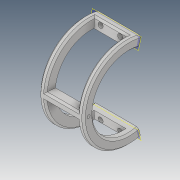
# Autodesk Inventor part: thrusterGuard2
Saved by Autodesk Inventor 2018 (Build 220112000, 112)
## iProperties
Created: 2020-01-11
Part Number: thrusterGuard2
Material: Generic
Document SubType Name: Modeling
Designer: anirudh
Density: 1 g/cm^3
Appearance: Default
Author: anirudh
Autodesk Inventor part; units mm, degrees
ref_plane "YZ Plane" through (0, 0, 0) normal (1, 0, 0) x (0, 1, 0)
ref_plane "XZ Plane" through (0, 0, 0) normal (0, 1, 0) x (-1, 0, 0)
ref_plane "XY Plane" through (0, 0, 0) normal (0, 0, 1) x (1, 0, 0)
sketch "Sketch1" plane through (0, 0, 0) normal (1, 0, 0) x (0, 1, 0)
  arc A0 (49.069, -13.148) -> (-49.069, -13.148) centre (0, 0) ccw
  arc A1 (62.7838, -16.8229) -> (-62.7838, -16.8229) centre (0, 0) ccw
  line L0 (49.069, -13.148) -> (62.7838, -16.8229)
  line L1 (0, 0) -> (80.3094, 0) construction
  line L2 (-49.069, -13.148) -> (-62.7838, -16.8229)
  line L3 (0, 0) -> (80.3094, 0) construction
  constraints: 8 end point, 4 point on circle, 2 centre point, 2 coincident, 2 horizontal
extrude "Extrusion1" add sketch "Sketch1" along normal blind 8.89
sketch "Sketch2" plane through (8.89, 0, 0) normal (1, 0, 0) x (0, 0, -1)
  line L0 (13.148, 49.069) -> (16.8229, 62.7838) projected
  line L1 (13.148, 49.069) -> (16.8229, 62.7838)
  arc A0 (16.8229, 62.7838) -> (16.8229, -62.7838) centre (0, 0) ccw projected
  line L2 (13.148, -49.069) -> (16.8229, -62.7838)
  line L3 (4.4275, 50.6067) -> (5.665, 64.7513)
  line L4 (0, 0) -> (73.6655, 0) construction
  line L5 (4.4275, -50.6067) -> (5.665, -64.7513)
  line L6 (0, 0) -> (73.6655, 0) construction
  line L7 (-50.6067, 4.4275) -> (-64.7513, 5.665)
  line L8 (0, 0) -> (70.0902, 0) construction
  line L9 (-50.6067, -4.4275) -> (-64.7513, -5.665)
  line L10 (0, 0) -> (70.0902, 0) construction
  arc A1 (16.8229, 62.7838) -> (5.665, 64.7513) centre (0, 0) ccw
  arc A2 (13.148, 49.069) -> (4.4275, 50.6067) centre (0, 0) ccw
  arc A3 (-50.6067, 4.4275) -> (-50.6067, -4.4275) centre (0, 0) ccw
  arc A4 (4.4275, -50.6067) -> (13.148, -49.069) centre (0, 0) ccw
  arc A5 (-64.7513, 5.665) -> (-64.7513, -5.665) centre (0, 0) ccw
  arc A6 (5.665, -64.7513) -> (16.8229, -62.7838) centre (0, 0) ccw
  dimension "d6" = 85
  dimension "d7" = 85
  dimension "d8" = 175
  dimension "d9" = 175
  constraints: 20 end point, 18 point on circle, 6 centre point, 4 horizontal, 2 coincident, 1 point on line
  measures "d6" angle of L4 L3
  measures "d7" angle of L5 L6
  measures "d8" angle of L8 L7
  measures "d9" angle of L9 L10
extrude "Extrusion2" add sketch "Sketch2" along normal blind 45.72
sketch "Sketch3" plane through (54.61, 0, 0) normal (1, 0, 0) x (0, 0, -1)
  line L0 (16.8229, 62.7838) -> (13.148, 49.069) projected
  arc A0 (16.8229, 62.7838) -> (16.8229, -62.7838) centre (0, 0) ccw
  arc A1 (13.148, 49.069) -> (13.148, -49.069) centre (0, 0) ccw
  line L1 (13.148, 49.069) -> (16.8229, 62.7838)
  arc A2 (16.8229, 62.7838) -> (16.8229, -62.7838) centre (0, 0) ccw projected
  arc A3 (13.148, 49.069) -> (13.148, -49.069) centre (0, 0) ccw projected
  line L2 (13.148, -49.069) -> (16.8229, -62.7838) projected
  line L3 (13.148, -49.069) -> (16.8229, -62.7838)
  constraints: 4 end point, 4 point on circle, 2 centre point, 2 coincident, 1 collinear
extrude "Extrusion3" add sketch "Sketch3" along normal blind 8.89
sketch "Sketch4" plane through (63.5, 62.7838, -16.8229) normal (0, -0.258819, -0.9659258) x (-1, 0, 0)
  line L0 (0, -115.7986) -> (0, -14.1986) projected
  line L1 (63.5, 0) -> (63.5, -14.1986) projected
  line L2 (63.5, 0) -> (63.5, -14.1986)
  line L3 (54.61, -14.9704) -> (54.61, -0.9875) projected
  circle A0 centre (17.78, -7.0993) radius 1.8
  circle A1 centre (45.72, -7.0993) radius 1.8
  point P0 (63.5, -64.9986)
  point P1 (0, 0)
  point P2 (0, -108.9927)
  dimension "d19" = 3.6
  dimension "d20" = 3.6
  constraints: 2 centre point, 2 end point, 1 vertical
  measures "d19" diameter of A0
  measures "d20" diameter of A1
extrude "Extrusion4" cut sketch "Sketch4" against normal blind 27.94
sketch "Sketch5" plane through (63.5, -49.069, -13.148) normal (0, 0.258819, -0.9659258) x (-1, 0, 0)
  line L0 (63.5, 0) -> (0, 0) projected
  line L1 (63.5, -14.1986) -> (0, -14.1986) projected
  line L2 (0, -14.1986) -> (0, 0) projected
  line L3 (63.5, 0) -> (63.5, -14.1986) projected
  circle A0 centre (17.78, -7.0993) radius 1.8
  circle A1 centre (45.72, -7.0993) radius 1.8
  point P0 (63.5, 50.8)
  dimension "d25" = 3.6
  dimension "d26" = 3.6
  constraints: 2 centre point
  measures "d25" diameter of A0
  measures "d26" diameter of A1
extrude "Extrusion5" cut sketch "Sketch5" against normal blind 27.94 contours A0 | A1
chamfer "Chamfer1" distance 2.54 angle 45 11 edges at (63.5, 0, 50.8) (63.5, 0, 64.9986) (8.89, 49.7918, 41.7803) (31.75, 64.7513, -5.665) (54.61, 49.7918, 41.7803) (31.75, 5.665, 64.7513) (8.89, -49.7918, 41.7803) (31.75, -5.665, 64.7513) (54.61, -49.7918, 41.7803) (0, 0, 64.9986) (0, 0, 50.8)
ref_plane "Work Plane1" through (60.96, 63.5603, -13.9251) normal (0, -0.258819, -0.9659258) x (-1, 0, 0)
sketch "Sketch8" plane through (60.96, 63.5603, -13.9251) normal (0, -0.258819, -0.9659258) x (-1, 0, 0)
  circle A0 centre (43.18, -7.0993) radius 1.8
  circle A1 centre (15.24, -7.0993) radius 3.6104
  line L0 (52.07, -3.4889) -> (6.35, -3.4889) projected
  circle A2 centre (43.18, -7.0993) radius 3.6104
  circle A3 centre (15.24, -7.0993) radius 3.6104
  point P0 (60.96, -64.9986)
  constraints: 4 centre point, 4 coincident, 2 tangent
extrude "Extrusion6" cut sketch "Sketch8" against normal blind 25.4 contours A0 | A1 | A2
ref_plane "Work Plane2" through (60.96, -49.8455, -10.2502) normal (0, 0.258819, -0.9659258) x (-1, 0, 0)
chamfer "Chamfer2" distance 2.54 angle 45 3 edges at (7.62, -64.7513, -5.665) (55.88, -64.7513, -5.665) (31.75, -64.7513, -5.665)
sketch "Sketch11" plane through (60.96, -49.8455, -10.2502) normal (0, 0.258819, -0.9659258) x (-1, 0, 0)
  circle A0 centre (43.18, -7.0993) radius 1.8 projected
  circle A1 centre (43.18, -7.0993) radius 3.6104
  line L0 (6.35, -10.7097) -> (52.07, -10.7097) projected
  circle A2 centre (15.24, -7.0993) radius 1.8 projected
  circle A3 centre (15.24, -7.0993) radius 3.611
  point P0 (60.96, 50.8)
  constraints: 2 centre point, 2 coincident, 1 tangent
extrude "Extrusion7" cut sketch "Sketch11" against normal blind 25.4 contours A0 | A1 | A2 | A3
sketch "Sketch12" plane through (0, 0, 0) normal (-1, 0, 0) x (0, 0, 1)
  arc A0 (-16.8229, -62.7838) -> (-16.8229, 62.7838) centre (0, 0) ccw projected
  arc A1 (-13.8054, -51.5225) -> (-13.8054, 51.5225) centre (0, 0) ccw projected
  line L0 (53.34, 0) -> (62.4586, 0)
  arc A2 (-16.1655, -60.3304) -> (-16.1655, 60.3304) centre (0, 0) ccw projected
  circle A3 centre (57.8993, 0) radius 2.2
  dimension "d41" = 4.4
  constraints: 2 end point, 2 point on circle, 1 centre point, 1 midpoint
  measures "d41" diameter of A3
extrude "Extrusion8" cut sketch "Sketch12" against normal blind 4.8
sketch "Sketch13" plane through (63.5, 0, 0) normal (1, 0, 0) x (0, 0, -1)
  arc A0 (16.8229, 62.7838) -> (16.8229, -62.7838) centre (0, 0) ccw projected
  arc A1 (16.1655, 60.3304) -> (16.1655, -60.3304) centre (0, 0) ccw projected
  arc A2 (13.8054, 51.5225) -> (13.8054, -51.5225) centre (0, 0) ccw projected
  circle A3 centre (-57.8993, 0) radius 2.2
  dimension "d44" = 4.4
  constraints: 1 centre point
  measures "d44" diameter of A3
extrude "Extrusion9" cut sketch "Sketch13" against normal blind 4.8
body "Solid1"
